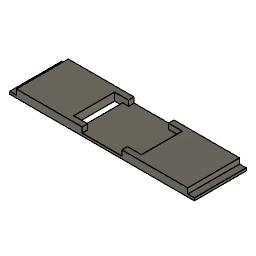
Canal - middle plate v3 (Autodesk Fusion 360 design; units mm, degrees)
Autodesk Fusion 360 part; units mm, degrees
sketch "Esquisse1" plane through (0, 0, 0) normal (0, 0, 1) x (1, 0, 0)
  line L0 (0.4, 40) -> (70, 40)
  line L1 (70, 40) -> (70, 20.4)
  line L2 (70, 20.4) -> (0.4, 20.4)
  line L3 (0.4, 20.4) -> (0.4, 40)
  dimension "d1" = 69.6
  dimension "d2" = 19.6
  constraint horizontal L0
  constraint vertical L1
  constraint horizontal L2
  constraint vertical L3
  measures "d1" distance of L1 L3
  measures "d2" distance of L0 L2
extrude "Extrusion1" add sketch "Esquisse1" along normal blind 3
sketch "Esquisse2" plane through (0, 0, 0) normal (0, 0, -1) x (1, 0, 0)
  line L0 (70, -20.4) -> (0.4, -20.4)
  line L1 (0.4, -20.4) -> (0.4, -40)
  line L2 (0.4, -40) -> (70, -40)
  line L3 (70, -40) -> (70, -20.4)
  line L4 (7.6, -22.3) -> (12.8, -22.3)
  line L5 (12.8, -22.3) -> (12.8, -24.5)
  line L6 (12.8, -24.5) -> (7.6, -24.5)
  line L7 (7.6, -24.5) -> (7.6, -22.3)
  line L8 (10.2, -22.3) -> (10.2, -24.5) construction
  line L9 (35.2, -20.4) -> (35.2, -40) construction
  line L10 (57.6, -22.3) -> (57.6, -24.5)
  line L11 (62.8, -22.3) -> (57.6, -22.3)
  line L12 (62.8, -24.5) -> (62.8, -22.3)
  line L13 (57.6, -24.5) -> (62.8, -24.5)
  line L14 (0.4, -30.2) -> (70, -30.2) construction
  line L15 (7.6, -38.1) -> (12.8, -38.1)
  line L16 (12.8, -38.1) -> (12.8, -35.9)
  line L17 (12.8, -35.9) -> (7.6, -35.9)
  line L18 (7.6, -35.9) -> (7.6, -38.1)
  line L19 (62.8, -38.1) -> (57.6, -38.1)
  line L20 (62.8, -35.9) -> (62.8, -38.1)
  line L21 (57.6, -35.9) -> (62.8, -35.9)
  line L22 (57.6, -38.1) -> (57.6, -35.9)
  dimension "d5" = 25
  dimension "d12" = 5.2
  dimension "d13" = 2.2
  dimension "d14" = 1.9
  constraint horizontal L4
  constraint vertical L5
  constraint horizontal L6
  constraint vertical L7
  constraint midpoint L4 L8.start
  constraint midpoint L6 L8.end
  constraint midpoint L0 L9.start
  constraint midpoint L2 L9.end
  constraint symmetric L4.start L9 L11.start
  constraint symmetric L4.end L9 L10.start
  constraint symmetric L5.end L9 L10.end
  constraint symmetric L6.end L9 L12.start
  constraint midpoint L1 L14.start
  constraint midpoint L3 L14.end
  constraint symmetric L4.start L14 L15.start
  constraint symmetric L4.end L14 L15.end
  constraint symmetric L5.end L14 L16.end
  constraint symmetric L6.end L14 L17.end
  constraint symmetric L10.start L14 L19.end
  constraint symmetric L10.end L14 L21.start
  constraint symmetric L11.start L14 L19.start
  constraint symmetric L12.start L14 L20.start
  measures "d5" distance of L8 L9
  measures "d12" distance of L5 L7
  measures "d13" distance of L4 L6
  measures "d14" distance of L0 L4
extrude "Extrusion2" cut sketch "Esquisse2" against normal blind 2 contours L4 L5 L6 L7 | L10 L11 L12 L13 | L15 L16 L17 L18 | L19 L20 L21 L22
sketch "Esquisse3" plane through (0, 0, 3) normal (0, 0, 1) x (-1, 0, 0)
  line L0 (-0.4, -20.4) -> (-70, -20.4)
  line L1 (-70, -20.4) -> (-70, -40)
  line L2 (-70, -40) -> (-0.4, -40)
  line L3 (-0.4, -40) -> (-0.4, -20.4)
  line L4 (-22.45, -37.9) -> (-47.95, -37.9)
  line L5 (-47.95, -37.9) -> (-47.95, -22.5)
  line L6 (-47.95, -22.5) -> (-22.45, -22.5)
  line L7 (-22.45, -22.5) -> (-22.45, -37.9)
  line L8 (-0.4, -30.2) -> (-70, -30.2) construction
  line L9 (-35.2, -40) -> (-35.2, -20.4) construction
  dimension "d8" = 25.5
  dimension "d9" = 15.4
  constraint horizontal L4
  constraint vertical L5
  constraint horizontal L6
  constraint vertical L7
  constraint midpoint L3 L8.start
  constraint midpoint L1 L8.end
  constraint midpoint L2 L9.start
  constraint midpoint L0 L9.end
  constraint symmetric L5 L7 L9
  constraint symmetric L0 L2 L8
  constraint symmetric L4 L6 L8
  measures "d8" distance of L5 L7
  measures "d9" distance of L4 L6
extrude "Extrusion3" cut sketch "Esquisse3" against normal blind 2 contours L4 L5 L6 L7
sketch "Esquisse4" plane through (0, 0, 1) normal (0, 0, 1) x (-1, 0, 0)
  line L0 (-22.45, -22.5) -> (-47.95, -22.5)
  line L1 (-47.95, -22.5) -> (-47.95, -37.9)
  line L2 (-47.95, -37.9) -> (-22.45, -37.9)
  line L3 (-22.45, -37.9) -> (-22.45, -22.5)
  line L4 (-22.45, -22.5) -> (-25.45, -22.5)
  line L5 (-25.45, -22.5) -> (-25.45, -37.9)
  line L6 (-25.45, -37.9) -> (-22.45, -37.9)
  line L7 (-22.45, -37.9) -> (-22.45, -22.5)
  dimension "d15" = 3
  constraint horizontal L4
  constraint vertical L5
  constraint horizontal L6
  constraint vertical L7
  constraint coincident L2 L5.end
  constraint coincident L0.start L3.end
  measures "d15" distance of L5 L7
extrude "Extrusion4" cut sketch "Esquisse4" against normal blind 3 contours L0 L2 L3 L4 L5 L6 L7
sketch "Esquisse5" plane through (0, 40, 0) normal (0, 1, 0) x (-1, 0, 0)
  line L0 (-70, 0) -> (-0.4, 0)
  line L1 (-0.4, 0) -> (-0.4, 3)
  line L2 (-0.4, 3) -> (-70, 3)
  line L3 (-70, 3) -> (-70, 0)
  line L4 (-35.2, 3) -> (-35.2, 0) construction
  line L5 (-42.7, 3) -> (-27.7, 3)
  line L6 (-27.7, 3) -> (-27.7, 1)
  line L7 (-27.7, 1) -> (-42.7, 1)
  line L8 (-42.7, 1) -> (-42.7, 3)
  dimension "d18" = 15
  dimension "d19" = 2
  constraint midpoint L2 L4.start
  constraint midpoint L0 L4.end
  constraint horizontal L5
  constraint vertical L6
  constraint horizontal L7
  constraint vertical L8
  constraint coincident L2 L5.start
  constraint symmetric L4 L6 L8
  measures "d18" distance of L6 L8
  measures "d19" distance of L5 L7
extrude "Extrusion5" cut sketch "Esquisse5" against normal blind 21 contours L2 L5 L6 L7 L8
sketch "Esquisse6" plane through (0, 0, 3) normal (0, 0, 1) x (-1, 0, 0)
  line L0 (-42.7, -22.5) -> (-42.7, -20.4)
  line L1 (-42.7, -20.4) -> (-70, -20.4)
  line L2 (-70, -20.4) -> (-70, -40)
  line L3 (-70, -40) -> (-42.7, -40)
  line L4 (-42.7, -40) -> (-42.7, -37.9)
  line L5 (-42.7, -37.9) -> (-47.95, -37.9)
  line L6 (-47.95, -37.9) -> (-47.95, -22.5)
  line L7 (-47.95, -22.5) -> (-42.7, -22.5)
  line L8 (-70, -40) -> (-67.5, -40)
  line L9 (-67.5, -40) -> (-67.5, -20.4)
  line L10 (-67.5, -20.4) -> (-70, -20.4)
  line L11 (-70, -20.4) -> (-70, -40)
  line L12 (-35.2, -39) -> (-35.2, -18) construction
  line L13 (-0.4, -20.4) -> (-0.4, -40)
  line L14 (-2.9, -20.4) -> (-0.4, -20.4)
  line L15 (-2.9, -40) -> (-2.9, -20.4)
  line L16 (-0.4, -40) -> (-2.9, -40)
  dimension "d22" = 2.5
  dimension "d23" = 34.8
  constraint horizontal L8
  constraint vertical L9
  constraint horizontal L10
  constraint vertical L11
  constraint coincident L1 L9.end
  constraint coincident L2.end L3.start
  constraint parallel L6 L12
  constraint symmetric L2.end L12 L13.end
  constraint symmetric L8.end L12 L15.start
  constraint symmetric L9.end L12 L14.start
  constraint symmetric L1.end L12 L13.start
  measures "d22" distance of L9 L11
  measures "d23" distance of L11 L12
extrude "Extrusion6" cut sketch "Esquisse6" against normal blind 2 contours L1 L2 L3 L8 L9 L10 L11 | L13 L14 L15 L16
